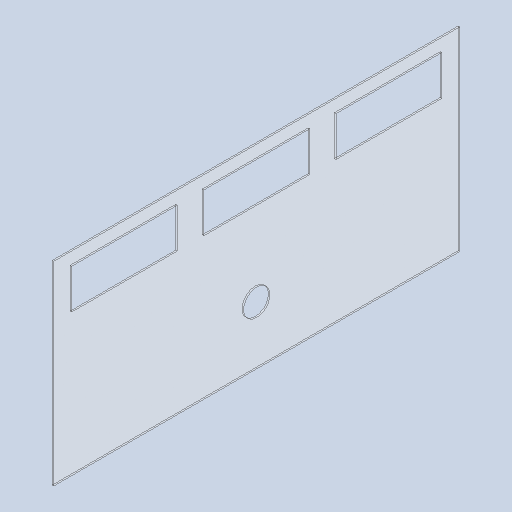
# Autodesk Inventor part: Posterior
Saved by Autodesk Inventor 2025.1 (Build 291241000, 241)
## iProperties
Created: 2024-09-06
Part Number: Posterior
Material: Acrylic
Document SubType Name: Modeling
Designer: joser
Density: 1.188 g/cm^3
Appearance: Transparent - Clear
Mass: 851.796 g
Surface Area: 4924.3 cm^2
Volume: 717 cm^3
Author: joser
Autodesk Inventor part; units mm, degrees
ref_plane "YZ Plane" through (0, 0, 0) normal (1, 0, 0) x (0, 1, 0)
ref_plane "XZ Plane" through (0, 0, 0) normal (0, 1, 0) x (-1, 0, 0)
ref_plane "XY Plane" through (0, 0, 0) normal (0, 0, 1) x (1, 0, 0)
sketch "Sketch1" plane through (0, 0, 0) normal (1, 0, 0) x (0, 1, 0)
  line L0 (-184, -384) -> (184, -384)
  line L1 (184, -384) -> (184, 384)
  line L2 (184, 384) -> (-184, 384)
  line L3 (-184, 384) -> (-184, -384)
  line L4 (-184, -384) -> (184, 384) construction
  line L5 (184, -384) -> (-184, 384) construction
  line L6 (159, 350) -> (84, 350)
  line L7 (84, 350) -> (84, 150)
  line L8 (84, 150) -> (159, 150)
  line L9 (159, 150) -> (159, 350)
  line L10 (159, -100) -> (159, 100)
  line L11 (159, 100) -> (84, 100)
  line L12 (84, 100) -> (84, -100)
  line L13 (84, -100) -> (159, -100)
  line L14 (159, -350) -> (159, -150)
  line L15 (159, -150) -> (84, -150)
  line L16 (84, -150) -> (84, -350)
  line L17 (84, -350) -> (159, -350)
  circle A0 centre (-75, 0) radius 25
  point P0 (0, 0)
  dimension "d0" = 768
  dimension "d1" = 368
  dimension "d2" = 200
  dimension "d3" = 75
  dimension "d4" = 34
  dimension "d5" = 25
  dimension "d8" = 250
  dimension "d17" = 75
  dimension "d18" = 50
  constraints: 36 end point, 4 parallel, 2 horizontal, 2 midpoint, 2 perpendicular, 1 centre point, 1 horizontal alignment, 1 vertical, 16 other
  measures "d0" distance of L0.end L1.end
  measures "d1" distance of L0.start L0.end
  measures "d2" distance of L8.end L6.start
  measures "d3" distance of L6.start L6.end
  measures "d4" distance between parallel lines of L2 L6
  measures "d5" distance between parallel lines of L9 L1
  measures "d8" distance of L8.end L10.start
  measures "d17" distance of A0.centre point (0, 0)
  measures "d18" diameter of A0
extrude "Extrusion1" add sketch "Sketch1" along normal mid plane 3
body "Solid1"
